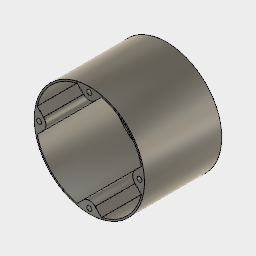
wall box v2 (Autodesk Fusion 360 design; units mm, degrees)
Autodesk Fusion 360 part; units mm, degrees
sketch "Sketch1" plane through (0, 0, 0) normal (0, 1, 0) x (1, 0, 0)
  circle A0 centre (0, 0) radius 30.5 construction
  circle A1 centre (0, -30.5) radius 1.5
  circle A2 centre (0, -30.5) radius 7.5 construction
  line L0 (-7.4123, -31.6434) -> (6.1101, -31.6434) construction
  line L1 (7.4123, -31.6434) -> (22.9663, -31.6434) construction
  line L2 (-7.4123, -31.6434) -> (-3.5355, -27.7667)
  line L3 (7.4123, -31.6434) -> (3.5355, -27.7667)
  arc A3 (3.5355, -27.7667) -> (-3.5355, -27.7667) centre (0, -31.3022) ccw
  circle A4 centre (0, 0) radius 33.5
  arc A5 (27.7667, 3.5355) -> (27.7667, -3.5355) centre (31.3022, 0) ccw
  line L4 (31.6434, -7.4123) -> (27.7667, -3.5355)
  line L5 (31.6434, 7.4123) -> (27.7667, 3.5355)
  circle A6 centre (30.5, 0) radius 1.5
  arc A7 (-3.5355, 27.7667) -> (3.5355, 27.7667) centre (0, 31.3022) ccw
  line L6 (7.4123, 31.6434) -> (3.5355, 27.7667)
  line L7 (-7.4123, 31.6434) -> (-3.5355, 27.7667)
  circle A8 centre (0, 30.5) radius 1.5
  arc A9 (-27.7667, -3.5355) -> (-27.7667, 3.5355) centre (-31.3022, 0) ccw
  line L8 (-31.6434, 7.4123) -> (-27.7667, 3.5355)
  line L9 (-31.6434, -7.4123) -> (-27.7667, -3.5355)
  circle A10 centre (-30.5, 0) radius 1.5
  arc A11 (7.4123, -31.6434) -> (31.6434, -7.4123) centre (0, 0) ccw
  arc A12 (31.6434, 7.4123) -> (7.4123, 31.6434) centre (0, 0) ccw
  arc A13 (-7.4123, 31.6434) -> (-31.6434, 7.4123) centre (0, 0) ccw
  arc A14 (-31.6434, -7.4123) -> (-7.4123, -31.6434) centre (0, 0) ccw
  dimension "d1" = 65
  dimension "d2" = 61
  dimension "d4" = 3
  dimension "d9" = 15
  dimension "d11" = 45
  dimension "d12" = 135
  dimension "d13" = 5
  dimension "d16" = 360
  measures "d1" diameter of A11
  measures "d2" diameter of A0
  measures "d4" diameter of A1
  measures "d9" diameter of A2
  measures "d11" angle of L0 L2
  measures "d12" angle of L1 L3
  measures "d13" radius of A3
extrude "Extrude1" add sketch "Sketch1" along normal blind 45
sketch "Sketch2" plane through (0, 45, 0) normal (0, 1, 0) x (-1, 0, 0)
  circle A0 centre (-30.5, 0) radius 1.5
  line L0 (31.6434, 7.4123) -> (27.7667, 3.5355)
  arc A1 (27.7667, 3.5355) -> (27.7667, -3.5355) centre (31.3022, 0) ccw
  line L1 (27.7667, -3.5355) -> (31.6434, -7.4123)
  arc A2 (7.4123, -31.6434) -> (31.6434, -7.4123) centre (0, 0) ccw
  line L2 (7.4123, -31.6434) -> (3.5355, -27.7667)
  arc A3 (3.5355, -27.7667) -> (-3.5355, -27.7667) centre (0, -31.3022) ccw
  line L3 (-3.5355, -27.7667) -> (-7.4123, -31.6434)
  arc A4 (-31.6434, -7.4123) -> (-7.4123, -31.6434) centre (0, 0) ccw
  line L4 (-31.6434, -7.4123) -> (-27.7667, -3.5355)
  arc A5 (-27.7667, -3.5355) -> (-27.7667, 3.5355) centre (-31.3022, 0) ccw
  line L5 (-27.7667, 3.5355) -> (-31.6434, 7.4123)
  arc A6 (-7.4123, 31.6434) -> (-31.6434, 7.4123) centre (0, 0) ccw
  line L6 (-7.4123, 31.6434) -> (-3.5355, 27.7667)
  arc A7 (-3.5355, 27.7667) -> (3.5355, 27.7667) centre (0, 31.3022) ccw
  line L7 (3.5355, 27.7667) -> (7.4123, 31.6434)
  arc A8 (31.6434, 7.4123) -> (7.4123, 31.6434) centre (0, 0) ccw
  circle A9 centre (0, 30.5) radius 1.5
  circle A10 centre (0, -30.5) radius 1.5
  circle A11 centre (30.5, 0) radius 1.5
  circle A12 centre (0, 0) radius 33.5
  circle A13 centre (0, 0) radius 33.5
extrude "Extrude2" add sketch "Sketch2" along normal blind 2 contours L0 A1 L1 A2 L2 A3 L3 A4 L4 A5 L5 A6 L6 A7 L7 A8 | A12 A13
